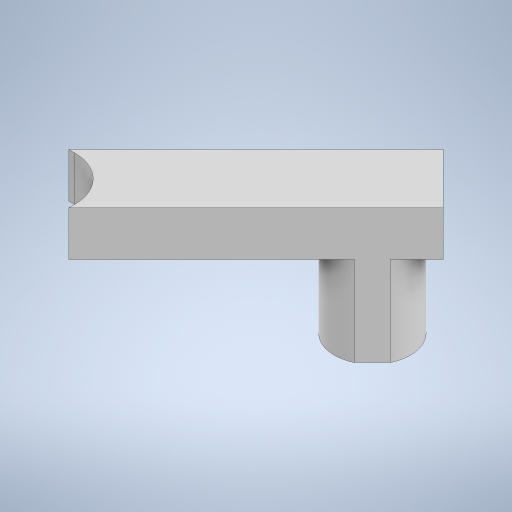
# Autodesk Inventor part: hjørner holder
Saved by Autodesk Inventor 2024 (Build 280153000, 153)
## iProperties
Created: 2024-03-15
Part Number: hjørner holder
Material: Generic
Document SubType Name: Modeling
Designer: laura
Density: 1 g/cm^3
Appearance: Default
Author: laura
Autodesk Inventor part; units mm, degrees
ref_plane "YZ Plane" through (0, 0, 0) normal (1, 0, 0) x (0, 1, 0)
ref_plane "XZ Plane" through (0, 0, 0) normal (0, 1, 0) x (-1, 0, 0)
ref_plane "XY Plane" through (0, 0, 0) normal (0, 0, 1) x (1, 0, 0)
sketch "Sketch1" plane through (0, 0, 0) normal (0, 1, 0) x (-1, 0, 0)
  circle A0 centre (28.3333, -28.3333) radius 8.5
  line L0 (56.6667, 0) -> (68, 0)
  line L1 (56.6667, 11.3333) -> (56.6667, 0)
  line L2 (68, 0) -> (26.0614, -41.9386)
  line L3 (68, 0) -> (127.3101, 0) construction
  line L4 (56.6667, 11.3333) -> (14.7281, -30.6053)
  line L5 (56.6667, 11.3333) -> (115.9768, 11.3333) construction
  line L6 (14.7281, -30.6053) -> (26.0614, -41.9386)
  point P0 (0, 0)
  point P1 (24.6701, -20.6632)
  point P2 (20.6632, -24.6701)
  point P3 (31.9965, -36.0035)
  point P4 (36.0035, -31.9965)
  dimension "d2" = 17
  dimension "d7" = 135
  dimension "d8" = 135
  constraints: 14 end point, 3 horizontal, 2 equal length, 1 centre point, 1 perpendicular
  measures "d2" diameter of A0
  measures "d7" angle of L2 L3
  measures "d8" angle of L4 L5
extrude "Extrusion1" add sketch "Sketch1" along normal blind 10 contours A0 L2 L4 | A0 L4 L1 L0 L2 | A0 L2 L6 L4
extrude "Extrusion2" add sketch "Sketch1" against normal blind 20 contours A0 L2 L4
fillet "Fillet1" radius 10 1 edges at (-56.6667, 5, 0)
body "Solid1"
